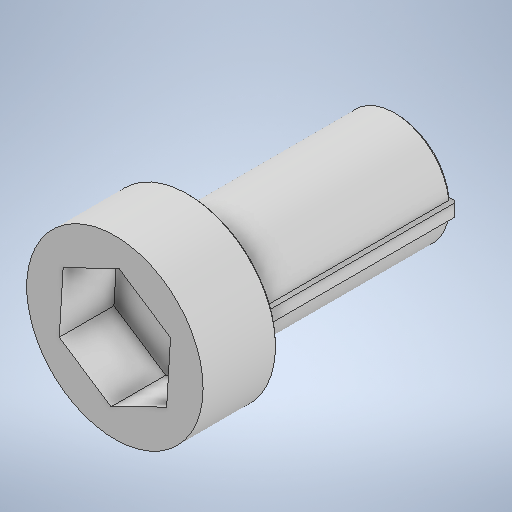
# Autodesk Inventor part: omni_ext
Saved by Autodesk Inventor 2025.1 (Build 291241000, 241)
## iProperties
Created: 2025-05-08
Part Number: omni_ext
Material: Generic
Document SubType Name: Modeling
Designer: User
Density: 1 g/cm^3
Appearance: Default
Author: User
## iProperties of the stored document omni_ext_3DPrint.ipt
Created: 2025-05-08
Part Number: omni_ext_3DPrint
Material: Generic
Document SubType Name: Modeling
Designer: User
Density: 1 g/cm^3
Appearance: Default
Author: User
Autodesk Inventor part; units mm, degrees
ref_plane "YZ Plane" through (0, 0, 0) normal (1, 0, 0) x (0, 1, 0)
ref_plane "XZ Plane" through (0, 0, 0) normal (0, 1, 0) x (-1, 0, 0)
ref_plane "Work Plane1" through (0, 0, 0) normal (0, 0, 1) x (1, 0, 0)
sketch "Sketch1" plane through (0, 0, 0) normal (0, 0, 1) x (1, 0, 0)
  line L0 (-9.8058, 6.0834) -> (-16.0096, 2.999) projected
  line L1 (-16.0096, 2.999) -> (-21.7826, 6.8295) projected
  line L2 (-21.7826, 6.8295) -> (-21.3519, 13.7443) projected
  line L3 (-21.3519, 13.7443) -> (-15.1481, 16.8286) projected
  line L4 (-15.1481, 16.8286) -> (-9.3751, 12.9982) projected
  line L5 (-9.3751, 12.9982) -> (-9.8058, 6.0834) projected
  line L6 (-15.1481, 16.8286) -> (-16.0096, 2.999)
  circle A0 centre (-15.5789, 9.9138) radius 10
  point P0 (0, 0)
  dimension "d0" = 12
  dimension "d1" = 20
  constraints: 2 end point, 1 centre point, 1 midpoint
  measures "d0" distance between parallel lines of L0 L3
  measures "d1" diameter of A0
extrude "Extrusion1" add sketch "Sketch1" against normal blind 6.2
sketch "Sketch2" plane through (-15.5789, 9.9138, -6.2) normal (0, 0, -1) x (-1, 0, 0)
  circle A0 centre (0, 0) radius 10 projected
  point P0 (-15.5789, -9.9138)
extrude "Extrusion2" add sketch "Sketch2" along normal blind 2.2
sketch "Sketch3" plane through (-15.5789, 9.9138, -8.4) normal (0, 0, -1) x (-1, 0, 0)
  circle A0 centre (0, 0) radius 10 projected
  circle A1 centre (0, 0) radius 3.3
  point P0 (-15.5789, -9.9138)
  dimension "d6" = 6.6
  constraints: 1 centre point, 1 coincident
  measures "d6" diameter of A1
extrude "Extrusion3" cut sketch "Sketch3" against normal through all contours A1
sketch "Sketch4" plane through (-15.5789, 9.9138, -8.4) normal (0, 0, -1) x (-1, 0, 0)
  circle A0 centre (0, 0) radius 3.3 projected
  circle A1 centre (0, 0) radius 6.1
  point P0 (-15.5789, -9.9138)
  dimension "d9" = 12.2
  constraints: 1 centre point, 1 coincident
  measures "d9" diameter of A1
extrude "Extrusion4" add sketch "Sketch4" along normal blind 23.5
chamfer "Chamfer3" distance 0.2 angle 45 1 edges at (-5.5789, 9.9138, -8.4)
sketch "Sketch6" plane through (-15.5789, 9.9138, -6.2) normal (0, 0, 1) x (1, 0, 0)
  circle A0 centre (0, 0) radius 3.3 projected
  point P0 (15.5789, -9.9138)
extrude "Extrusion6" add sketch "Sketch6" against normal blind 2.3
sketch "Sketch7" plane through (-15.5789, 9.9138, -8.5) normal (0, 0, -1) x (-1, 0, 0)
  circle A0 centre (0, 0) radius 3.3 projected
  circle A1 centre (0, 0) radius 1.92
  point P0 (-15.5789, -9.9138)
  dimension "d42" = 3.84
  constraints: 1 centre point, 1 coincident
  measures "d42" diameter of A1
extrude "Extrusion7" cut sketch "Sketch7" against normal through all contours A1
sketch "Sketch9" plane through (-15.5789, 9.9138, -6.2) normal (0, 0, 1) x (1, 0, 0)
  circle A0 centre (0, 0) radius 1.92 projected
  circle A1 centre (0, 0) radius 2.02
  point P0 (15.5789, -9.9138)
  dimension "d52" = 0.1
  constraints: 1 centre point
  measures "d52" radial gap between concentric circles of A0 A1
extrude "Extrusion8" cut sketch "Sketch9" against normal blind 10 contours A0 | A1
sketch "Sketch10" plane through (-15.5789, 9.9138, 0) normal (0, 0, 1) x (1, 0, 0)
  circle A0 centre (0, 0) radius 10 projected
  line L0 (0.4308, 6.9148) -> (6.2038, 3.0844) projected
  line L1 (6.2038, 3.0844) -> (5.773, -3.8304) projected
  line L2 (5.773, -3.8304) -> (-0.4308, -6.9148) projected
  line L3 (-0.4308, -6.9148) -> (-6.2038, -3.0844) projected
  line L4 (-6.2038, -3.0844) -> (-5.773, 3.8304) projected
  line L5 (-5.773, 3.8304) -> (0.4308, 6.9148) projected
  line L6 (5.8692, -3.8943) -> (6.3072, 3.1358)
  line L7 (6.3072, 3.1358) -> (0.4379, 7.03)
  line L8 (0.4379, 7.03) -> (-5.8692, 3.8943)
  line L9 (-5.8692, 3.8943) -> (-6.3072, -3.1358)
  line L10 (-6.3072, -3.1358) -> (-0.4379, -7.03)
  line L11 (-0.4379, -7.03) -> (5.8692, -3.8943)
  point P0 (15.5789, -9.9138)
  dimension "d55" = 0.1
  constraints: 12 end point, 5 other
  measures "d55" distance between parallel lines of L1 L6
extrude "Extrusion9" cut sketch "Sketch10" against normal up to surface (6.2 mm away) contours L11 L10 L9 L8 L7 L6
thicken "Thicken3" operation add thickness 0.1 both sides no extend neighbours no toward (0, 0, -1) faces at (-20.6545, 9.164, -31.9) (-21.6591, 9.423, -24.0667)
sketch "Sketch11" plane through (-15.5789, 9.9138, -32) normal (0, 0, -1) x (-1, 0, 0)
  circle A0 centre (0, 0) radius 6.2 projected
  circle A1 centre (0, 0) radius 6.2 projected
  line L0 (-6.2, 0) -> (-6.2, 0.7)
  line L1 (-6.2, 0) -> (-5.5, 0) construction
  line L2 (-6.2, 0) -> (-6.2, -0.7)
  line L3 (-6.2, 0) -> (-5.5, 0) construction
  line L4 (-6.2, 0) -> (-6.7, 0)
  line L5 (-6.75, -0.7) -> (-5.75, -0.7)
  line L6 (-5.75, -0.7) -> (-5.75, 0.7)
  line L7 (-5.75, 0.7) -> (-6.75, 0.7)
  line L8 (-6.75, 0.7) -> (-6.75, -0.7)
  point P0 (-15.5789, -9.9138)
  dimension "d60" = 0.7
  dimension "d61" = 90
  dimension "d62" = 0.7
  dimension "d63" = 90
  dimension "d64" = 0.5
  dimension "d79" = 1
  dimension "d80" = 5.75
  constraints: 18 end point, 3 horizontal, 3 perpendicular, 2 parallel, 2 vertical, 1 horizontal alignment, 1 point on line, 1 tangent, 1 other
  measures "d60" distance of L0.start L0.end
  measures "d61" angle of L1 L0
  measures "d62" distance of L0.start L2.end
  measures "d63" angle of L2 L3
  measures "d64" distance of L0.start L4.end
  measures "d79" distance of L6.end L7.end
  measures "d80" distance from line of L6 A0.centre
extrude "Extrusion10" add sketch "Sketch11" against normal up to surface (23.6 mm away) contours L7 L6 L5 A0 | A0 L0 L7 | L5 L2 A0 | L2 L5 L8 L7 L0 picked at (-5.9, 0)
chamfer "Chamfer9" distance 0.3 angle 45 2 edges at (-15.9294, 3.7237, -32) (-15.9294, 16.1039, -32)
chamfer "Chamfer10" distance 0.3 angle 45 1 edges at (-8.8289, 9.9138, -32)
sketch "Sketch14" plane through (-15.5789, 9.9138, -32) normal (0, 0, -1) x (-1, 0, 0)
  line L0 (-6.45, -0.7) -> (-6.45, 0.7) projected
  line L1 (-6.45, -0.7) -> (-5.8583, -0.7) projected
  arc A0 (-5.8583, -0.7) -> (-5.8583, 0.7) centre (0, 0) ccw projected
  line L2 (-5.8583, 0.7) -> (-6.45, 0.7) projected
  circle A1 centre (0, 0) radius 3.3 projected
  circle A2 centre (0, 0) radius 3.95
  point P0 (-15.5789, -9.9138)
  dimension "d75" = 6.6
  dimension "d76" = 7.9
  constraints: 1 centre point, 1 coincident
  measures "d75" diameter of A1
  measures "d76" diameter of A2
extrude "Extrusion12" cut sketch "Sketch14" against normal up to surface (23.5 mm away) contours A1 | A2
body "Solid1"
